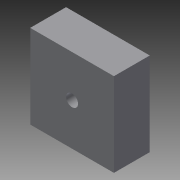
# Autodesk Inventor part: tension_block
Saved by Autodesk Inventor 2015 SP1 (Build 190203100, 203)
## iProperties
Created: 2014-12-28
Part Number: tension_block
Material: Generic
Document SubType Name: Modeling
Designer: Jarod
Density: 1 g/cm^3
Appearance: Default
Author: Jarod
Autodesk Inventor part; units mm, degrees
ref_plane "YZ Plane" through (0, 0, 0) normal (1, 0, 0) x (0, 1, 0)
ref_plane "XZ Plane" through (0, 0, 0) normal (0, 1, 0) x (-1, 0, 0)
ref_plane "XY Plane" through (0, 0, 0) normal (0, 0, 1) x (1, 0, 0)
sketch "Sketch1" plane through (0, 0, 0) normal (1, 0, 0) x (0, 1, 0)
  line L0 (0, 0) -> (44.45, 0)
  line L1 (44.45, 0) -> (44.45, -19.05)
  line L2 (44.45, -19.05) -> (0, -19.05)
  line L3 (0, -19.05) -> (0, 0)
  dimension "d0" = 44.45
  dimension "d1" = 19.05
  constraints: 8 end point, 2 parallel, 1 horizontal, 1 perpendicular
  measures "d0" distance of L1.end L2.end
  measures "d1" distance of L0.end L1.end
extrude "Extrusion1" add sketch "Sketch1" along normal blind 44.45
sketch "Sketch2" plane through (0, 0, 0) normal (0, 0, 1) x (1, 0, 0)
  line L0 (0, 0) -> (0, 44.45) projected
  line L1 (0, 0) -> (44.45, 0) projected
  line L2 (44.45, 44.45) -> (44.45, 0) projected
  line L3 (0, 44.45) -> (44.45, 44.45) projected
  point P0 (22.225, 22.225)
  dimension "d4" = 22.225
  dimension "d5" = 22.225
  measures "d4" distance from line of L0 point (22.225, 22.225)
  measures "d5" distance from line of L1 point (22.225, 22.225)
hole "Hole1" at (22.225, 22.225, 0) direction (0, 0, -1) diameter 6.35 end through all
body "Solid1"
